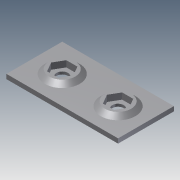
# Autodesk Inventor part: bracket_plastictube
Saved by Autodesk Inventor 2011 (Build 150239000, 239)
## iProperties
Created: 2012-11-30
Part Number: bracket_plastictube
Document SubType Name: Modeling
Designer: Administrator
Density: 1 g/cm^3
Author: Administrator
Autodesk Inventor part; units mm, degrees
ref_plane "YZ Plane" through (0, 0, 0) normal (1, 0, 0) x (0, 1, 0)
ref_plane "XZ Plane" through (0, 0, 0) normal (0, 1, 0) x (-1, 0, 0)
ref_plane "XY Plane" through (0, 0, 0) normal (0, 0, 1) x (1, 0, 0)
sketch "Sketch4" plane through (0, 0, 0) normal (0, 0, 1) x (1, 0, 0)
  line L0 (-21.5, 10.75) -> (0, 10.75)
  line L1 (0, 10.75) -> (0, -10.75)
  line L2 (0, -10.75) -> (-21.5, -10.75)
  line L3 (-21.5, -10.75) -> (-21.5, 10.75)
  circle A0 centre (-10.75, 0) radius 2.2
  point P0 (0, 0)
  point P1 (-21.5, 0)
  point P2 (0, 0)
  point P3 (-10.75, 10.75)
  dimension "d12" = 21.5
  dimension "d13" = 21.5
  dimension "d14" = 4.4
  constraints: 8 end point, 3 midpoint, 2 horizontal alignment, 2 parallel, 2 vertical alignment, 1 centre point, 1 horizontal, 1 perpendicular
  measures "d12" distance of L0.start L0.end
  measures "d13" distance of L2.end L0.start
  measures "d14" diameter of A0
extrude "Extrusion4" add sketch "Sketch4" along normal blind 1.75
sketch "Sketch5" plane through (0, 0, 1.75) normal (0, 0, 1) x (1, 0, 0)
  circle A0 centre (-10.75, 0) radius 2.2 projected
  circle A1 centre (-10.75, 0) radius 6.7
  point P0 (0, 0)
  dimension "d17" = 13.4
  constraints: 1 centre point, 1 coincident
  measures "d17" diameter of A1
extrude "Extrusion5" add sketch "Sketch5" along normal blind 1.65
draft "FaceDraft2" angle 45 pull direction (0, 0, 1) faces at (-4.1368, -1.0748, 2.85) fixed edges at (-17.45, 0, 1.75)
sketch "Sketch6" plane through (-10.75, 0, 3.4) normal (0, 0, 1) x (1, 0, 0)
  circle A0 centre (0, 0) radius 2.2 projected
  circle A1 centre (0, 0) radius 5.05 projected
  line L0 (2.1362, -3.7) -> (-2.1362, -3.7)
  line L1 (-2.1362, -3.7) -> (-4.2724, 0)
  line L2 (-4.2724, 0) -> (-2.1362, 3.7)
  line L3 (-2.1362, 3.7) -> (2.1362, 3.7)
  line L4 (2.1362, 3.7) -> (4.2724, 0)
  line L5 (4.2724, 0) -> (2.1362, -3.7)
  line L6 (-10.75, 10.75) -> (10.75, 10.75) projected
  point P0 (10.75, 0)
  dimension "d21" = 7.4
  constraints: 12 end point, 1 coincident, 1 parallel, 13 other
  measures "d21" distance between parallel lines of L0 L3
extrude "Extrusion6" cut sketch "Sketch6" against normal blind 2.4 contours L0 L1 L2 L3 L4 L5
mirror "Mirror1" about plane through (0, 10.75, 0) normal (1, 0, 0) of "Extrusion4", "FaceDraft2", "Extrusion5", "Extrusion6"
body "Solid2"
